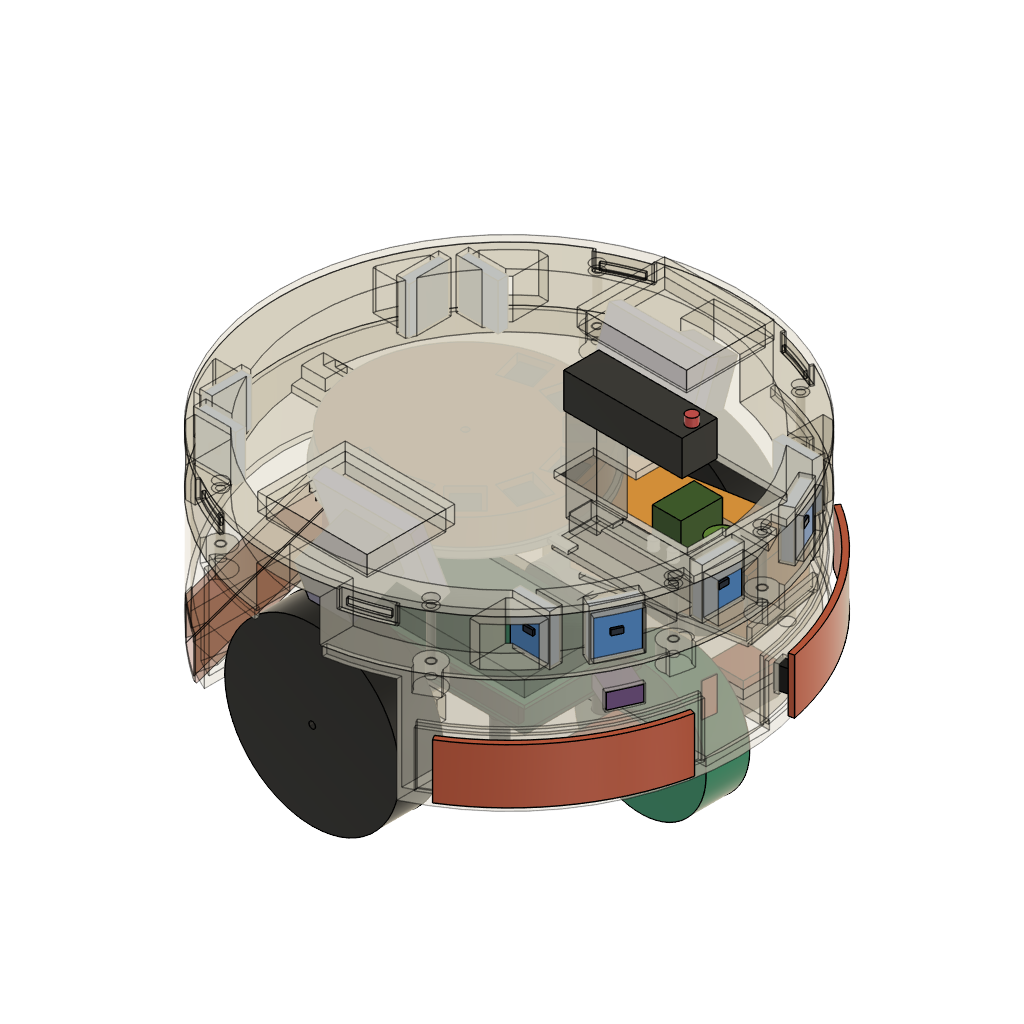
Theseus_V3_rev4 (Autodesk Fusion 360 design; units mm, degrees)
Autodesk Fusion 360 part; units mm, degrees
(part 1 of 3)
sketch "Tub shell sketch" plane through (0, 0, 0) normal (0, 0, 1) x (1, 0, 0) in component "Tub"
  circle A0 centre (0, 0) radius 105
extrude "Tub shell" add sketch "Tub shell sketch" along normal blind 52 from surface at 35 makes body 1 in component "Tub"
sketch "Cavity sketch" plane through (0, 0, 0) normal (0, 0, 1) x (1, 0, 0) in component "Tub"
  circle A0 centre (0, 0) radius 103
extrude "Cavity" cut sketch "Cavity sketch" along normal blind 53 from surface at 39 bodies 1 in component "Tub"
sketch "Rear chamfer sketch" plane through (0, 0, 0) normal (0, 1, 0) x (1, 0, 0) in component "Tub"
  line L0 (-65, -35) -> (-112, -56.15)
  line L1 (-112, -56.15) -> (-112, -29)
  line L2 (-112, -29) -> (-65, -29)
  line L3 (-65, -29) -> (-65, -35)
extrude "Rear chamfer" cut sketch "Rear chamfer sketch" along normal blind 220 from surface at -110 bodies 1 in component "Tub"
sketch "Wheel opening and arch L sketch" plane through (0, 0, 0) normal (0, 0, 1) x (1, 0, 0) in component "Tub"
  line L0 (-44, 69) -> (44, 69)
  line L1 (44, 69) -> (44, 108)
  line L2 (44, 108) -> (-44, 108)
  line L3 (-44, 108) -> (-44, 69)
extrude "Wheel opening and arch L" cut sketch "Wheel opening and arch L sketch" along normal blind 49 from surface at 34 bodies 1 in component "Tub"
sketch "Camera notch L sketch" plane through (0, 0, 0) normal (0, 0, 1) x (1, 0, 0) in component "Tub"
  line L0 (-11.9288, 69) -> (18.0712, 69)
  line L1 (18.0712, 69) -> (18.0712, 108)
  line L2 (18.0712, 108) -> (-11.9288, 108)
  line L3 (-11.9288, 108) -> (-11.9288, 69)
extrude "Camera notch L" cut sketch "Camera notch L sketch" along normal blind 6 from surface at 82 bodies 1 in component "Tub"
sketch "Motor seat L sketch" plane through (0, 0, 0) normal (0, 1, 0) x (1, 0, 0) in component "Tub"
  circle A0 centre (0, -40) radius 10.15
extrude "Motor seat L" cut sketch "Motor seat L sketch" along normal blind 51.5 from surface at 13 bodies 1 in component "Tub"
sketch "Shaft notch L sketch" plane through (0, 0, 0) normal (0, 1, 0) x (1, 0, 0) in component "Tub"
  line L0 (-3, -34.5) -> (3, -34.5)
  line L1 (3, -34.5) -> (3, -44.5)
  line L2 (3, -44.5) -> (-3, -44.5)
  line L3 (-3, -44.5) -> (-3, -34.5)
extrude "Shaft notch L" cut sketch "Shaft notch L sketch" along normal blind 4.5 from surface at 64.5 bodies 1 in component "Tub"
sketch "Plate slot L sketch" plane through (0, 0, 0) normal (0, 0, 1) x (1, 0, 0) in component "Tub"
  line L0 (-16, 60.5) -> (24.5, 60.5)
  line L1 (24.5, 60.5) -> (24.5, 64.5)
  line L2 (24.5, 64.5) -> (-16, 64.5)
  line L3 (-16, 64.5) -> (-16, 60.5)
extrude "Plate slot L" cut sketch "Plate slot L sketch" along normal blind 5 from surface at 34.5 bodies 1 in component "Tub"
sketch "Wheel opening and arch R sketch" plane through (0, 0, 0) normal (0, 0, 1) x (1, 0, 0) in component "Tub"
  line L0 (-44, -108) -> (44, -108)
  line L1 (44, -108) -> (44, -69)
  line L2 (44, -69) -> (-44, -69)
  line L3 (-44, -69) -> (-44, -108)
extrude "Wheel opening and arch R" cut sketch "Wheel opening and arch R sketch" along normal blind 49 from surface at 34 bodies 1 in component "Tub"
sketch "Camera notch R sketch" plane through (0, 0, 0) normal (0, 0, 1) x (1, 0, 0) in component "Tub"
  line L0 (-11.9288, -108) -> (18.0712, -108)
  line L1 (18.0712, -108) -> (18.0712, -69)
  line L2 (18.0712, -69) -> (-11.9288, -69)
  line L3 (-11.9288, -69) -> (-11.9288, -108)
extrude "Camera notch R" cut sketch "Camera notch R sketch" along normal blind 6 from surface at 82 bodies 1 in component "Tub"
sketch "Motor seat R sketch" plane through (0, 0, 0) normal (0, 1, 0) x (1, 0, 0) in component "Tub"
  circle A0 centre (0, -40) radius 10.15
extrude "Motor seat R" cut sketch "Motor seat R sketch" along normal blind 51.5 from surface at -64.5 bodies 1 in component "Tub"
sketch "Shaft notch R sketch" plane through (0, 0, 0) normal (0, 1, 0) x (1, 0, 0) in component "Tub"
  line L0 (-3, -34.5) -> (3, -34.5)
  line L1 (3, -34.5) -> (3, -44.5)
  line L2 (3, -44.5) -> (-3, -44.5)
  line L3 (-3, -44.5) -> (-3, -34.5)
extrude "Shaft notch R" cut sketch "Shaft notch R sketch" along normal blind 4.5 from surface at -69 bodies 1 in component "Tub"
sketch "Plate slot R sketch" plane through (0, 0, 0) normal (0, 0, 1) x (1, 0, 0) in component "Tub"
  line L0 (-16, -64.5) -> (24.5, -64.5)
  line L1 (24.5, -64.5) -> (24.5, -60.5)
  line L2 (24.5, -60.5) -> (-16, -60.5)
  line L3 (-16, -60.5) -> (-16, -64.5)
extrude "Plate slot R" cut sketch "Plate slot R sketch" along normal blind 5 from surface at 34.5 bodies 1 in component "Tub"
sketch "Omni bay 1 sketch" plane through (0, 0, 0) normal (0, 1, 0) x (1, 0, 0) in component "Tub"
  line L0 (38.5005, -29.8229) -> (38.4302, -42.3229)
  arc A0 (38.4302, -42.3229) -> (101.4292, -42.6771) centre (69.9297, -42.5) ccw
  line L1 (101.4292, -42.6771) -> (101.4995, -30.1771)
  arc A1 (101.4995, -30.1771) -> (38.5005, -29.8229) centre (70, -30) ccw
extrude "Omni bay 1" cut sketch "Omni bay 1 sketch" along normal blind 29 from surface at -11.5 bodies 1 in component "Tub"
sketch "Omni bay 2 sketch" plane through (0, 0, 0) normal (0, 1, 0) x (1, 0, 0) in component "Tub"
  line L0 (39.7548, -33.4597) -> (36.0099, -45.9597)
  arc A0 (36.0099, -45.9597) -> (96.3596, -64.0403) centre (66.1848, -55) ccw
  line L1 (96.3596, -64.0403) -> (100.1046, -51.5403)
  arc A1 (100.1046, -51.5403) -> (39.7548, -33.4597) centre (69.9297, -42.5) ccw
extrude "Omni bay 2" cut sketch "Omni bay 2 sketch" along normal blind 29 from surface at -11.5 bodies 1 in component "Tub"
sketch "Arm slot sketch" plane through (0, 0, 0) normal (0, 1, 0) x (1, 0, 0) in component "Tub"
  line L0 (26.569, -43.9283) -> (71.069, -37.9283)
  arc A0 (71.069, -37.9283) -> (68.931, -22.0717) centre (70, -30) ccw
  line L1 (68.931, -22.0717) -> (24.431, -28.0717)
  arc A1 (24.431, -28.0717) -> (26.569, -43.9283) centre (25.5, -36) ccw
extrude "Arm slot" cut sketch "Arm slot sketch" along normal blind 9 from surface at 8.5 bodies 1 in component "Tub"
sketch "Floor port FP hole sketch" plane through (0, 0, 0) normal (0, 0, 1) x (1, 0, 0) in component "Tub"
  line L0 (66.5, 23.5) -> (83.5, 23.5)
  line L1 (83.5, 23.5) -> (83.5, 40.5)
  line L2 (83.5, 40.5) -> (66.5, 40.5)
  line L3 (66.5, 40.5) -> (66.5, 23.5)
extrude "Floor port FP hole" cut sketch "Floor port FP hole sketch" along normal blind 6 from surface at 34 bodies 1 in component "Tub"
sketch "Silver module SM hole sketch" plane through (0, 0, 0) normal (0, 0, 1) x (1, 0, 0) in component "Tub"
  line L0 (64.5, -38.5) -> (85.5, -38.5)
  line L1 (85.5, -38.5) -> (85.5, -15.5)
  line L2 (85.5, -15.5) -> (64.5, -15.5)
  line L3 (64.5, -15.5) -> (64.5, -38.5)
extrude "Silver module SM hole" cut sketch "Silver module SM hole sketch" along normal blind 6 from surface at 34 bodies 1 in component "Tub"
sketch "Chute hole tool B left sketch" plane through (0, 0, 0) normal (0, 0, 1) x (1, 0, 0) in component "Tub"
  line L0 (-8.5, -8.5) -> (8.5, -8.5)
  line L1 (8.5, -8.5) -> (8.5, 8.5)
  line L2 (8.5, 8.5) -> (-8.5, 8.5)
  line L3 (-8.5, 8.5) -> (-8.5, -8.5)
extrude "Chute hole tool B left" add sketch "Chute hole tool B left sketch" along normal blind 79.2151 separate body makes body 2 in component "Tub"
move_body "Move1" bodies 2 to x (-0.977496, -0.210954, 0) y (-0.112564, 0.521586, 0.845741) z (-0.178413, 0.826708, -0.533594) at (-47.2943, 27.2943, 79.5) in component "Tub"
combine "Combine1" operation cut target body 1 tool bodies 2 in component "Tub"
sketch "Chute hole tool A right sketch" plane through (0, 0, 0) normal (0, 0, 1) x (1, 0, 0) in component "Tub"
  line L0 (-8.5, -8.5) -> (8.5, -8.5)
  line L1 (8.5, -8.5) -> (8.5, 8.5)
  line L2 (8.5, 8.5) -> (-8.5, 8.5)
  line L3 (-8.5, 8.5) -> (-8.5, -8.5)
extrude "Chute hole tool A right" add sketch "Chute hole tool A right sketch" along normal blind 79.2151 separate body makes body 3 in component "Tub"
move_body "Move2" bodies 3 to x (0.977496, -0.210954, 0) y (-0.112564, -0.521586, 0.845741) z (-0.178413, -0.826708, -0.533594) at (-47.2943, -27.2943, 79.5) in component "Tub"
combine "Combine2" operation cut target body 1 tool bodies 3 in component "Tub"
sketch "Bumper recess L sketch" plane through (0, 0, 0) normal (0, 0, 1) x (1, 0, 0) in component "Tub"
  arc A0 (106.949, 15.0307) -> (50.7029, 95.3583) centre (0, 0) ccw
  line L0 (50.7029, 95.3583) -> (48.5903, 91.3851)
  arc A1 (102.4927, 14.4044) -> (48.5903, 91.3851) centre (0, 0) ccw
  line L1 (102.4927, 14.4044) -> (106.949, 15.0307)
extrude "Bumper recess L" cut sketch "Bumper recess L sketch" along normal blind 25 from surface at 40 bodies 1 in component "Tub"
sketch "Bumper recess wall L sketch" plane through (0, 0, 0) normal (0, 0, 1) x (1, 0, 0) in component "Tub"
  arc A0 (102.1957, 14.3627) -> (48.4495, 91.1202) centre (0, 0) ccw
  line L0 (48.4495, 91.1202) -> (47.6514, 89.6192)
  arc A1 (100.5122, 14.1261) -> (47.6514, 89.6192) centre (0, 0) ccw
  line L1 (100.5122, 14.1261) -> (102.1957, 14.3627)
extrude "Bumper recess wall L" add sketch "Bumper recess wall L sketch" along normal blind 27 from surface at 39 bodies 1 in component "Tub"
sketch "Bumper switch pocket L sketch" plane through (0, 0, 0) normal (0, 0, 1) x (1, 0, 0) in component "Tub"
  line L0 (98.18, 21.6448) -> (101.576, 22.4916)
  line L1 (101.576, 22.4916) -> (100.2455, 27.8282)
  line L2 (100.2455, 27.8282) -> (96.8494, 26.9815)
  line L3 (96.8494, 26.9815) -> (98.18, 21.6448)
extrude "Bumper switch pocket L" cut sketch "Bumper switch pocket L sketch" along normal blind 12 from surface at 46.5 bodies 1 in component "Tub"
sketch "Bumper recess R sketch" plane through (0, 0, 0) normal (0, 0, 1) x (1, 0, 0) in component "Tub"
  arc A0 (50.7029, -95.3583) -> (106.949, -15.0307) centre (0, 0) ccw
  line L0 (106.949, -15.0307) -> (102.4927, -14.4044)
  arc A1 (48.5903, -91.3851) -> (102.4927, -14.4044) centre (0, 0) ccw
  line L1 (48.5903, -91.3851) -> (50.7029, -95.3583)
extrude "Bumper recess R" cut sketch "Bumper recess R sketch" along normal blind 25 from surface at 40 bodies 1 in component "Tub"
sketch "Bumper recess wall R sketch" plane through (0, 0, 0) normal (0, 0, 1) x (1, 0, 0) in component "Tub"
  arc A0 (48.4495, -91.1202) -> (102.1957, -14.3627) centre (0, 0) ccw
  line L0 (102.1957, -14.3627) -> (100.5122, -14.1261)
  arc A1 (47.6514, -89.6192) -> (100.5122, -14.1261) centre (0, 0) ccw
  line L1 (47.6514, -89.6192) -> (48.4495, -91.1202)
extrude "Bumper recess wall R" add sketch "Bumper recess wall R sketch" along normal blind 27 from surface at 39 bodies 1 in component "Tub"
sketch "Bumper switch pocket R sketch" plane through (0, 0, 0) normal (0, 0, 1) x (1, 0, 0) in component "Tub"
  line L0 (96.8494, -26.9815) -> (100.2455, -27.8282)
  line L1 (100.2455, -27.8282) -> (101.576, -22.4916)
  line L2 (101.576, -22.4916) -> (98.18, -21.6448)
  line L3 (98.18, -21.6448) -> (96.8494, -26.9815)
extrude "Bumper switch pocket R" cut sketch "Bumper switch pocket R sketch" along normal blind 12 from surface at 46.5 bodies 1 in component "Tub"
sketch "Insert boss +12 sketch" plane through (0, 0, 0) normal (0, 0, 1) x (1, 0, 0) in component "Tub"
  circle A0 centre (95.3694, 20.2714) radius 6
  line L0 (96.4089, 15.3807) -> (102.7669, 16.7321)
  line L1 (102.7669, 16.7321) -> (100.6878, 26.5136)
  line L2 (100.6878, 26.5136) -> (94.3298, 25.1621)
  line L3 (94.3298, 25.1621) -> (96.4089, 15.3807)
extrude "Insert boss +12" add sketch "Insert boss +12 sketch" along normal blind 10 from surface at 77 bodies 1 in component "Tub"
sketch "Insert boss +60 sketch" plane through (0, 0, 0) normal (0, 0, 1) x (1, 0, 0) in component "Tub"
  circle A0 centre (48.75, 84.4375) radius 6
  line L0 (53.0801, 81.9375) -> (56.3301, 87.5666)
  line L1 (56.3301, 87.5666) -> (47.6699, 92.5666)
  line L2 (47.6699, 92.5666) -> (44.4199, 86.9375)
  line L3 (44.4199, 86.9375) -> (53.0801, 81.9375)
extrude "Insert boss +60" add sketch "Insert boss +60 sketch" along normal blind 10 from surface at 77 bodies 1 in component "Tub"
sketch "Insert boss +118 sketch" plane through (0, 0, 0) normal (0, 0, 1) x (1, 0, 0) in component "Tub"
  circle A0 centre (-45.7735, 86.0874) radius 6
  line L0 (-41.3587, 88.4347) -> (-44.4103, 94.1739)
  line L1 (-44.4103, 94.1739) -> (-53.2398, 89.4792)
  line L2 (-53.2398, 89.4792) -> (-50.1882, 83.74)
  line L3 (-50.1882, 83.74) -> (-41.3587, 88.4347)
extrude "Insert boss +118" add sketch "Insert boss +118 sketch" along normal blind 10 from surface at 77 bodies 1 in component "Tub"
sketch "Insert boss -12 sketch" plane through (0, 0, 0) normal (0, 0, 1) x (1, 0, 0) in component "Tub"
  circle A0 centre (95.3694, -20.2714) radius 6
  line L0 (94.3298, -25.1621) -> (100.6878, -26.5136)
  line L1 (100.6878, -26.5136) -> (102.7669, -16.7321)
  line L2 (102.7669, -16.7321) -> (96.4089, -15.3807)
  line L3 (96.4089, -15.3807) -> (94.3298, -25.1621)
extrude "Insert boss -12" add sketch "Insert boss -12 sketch" along normal blind 10 from surface at 77 bodies 1 in component "Tub"
sketch "Insert boss -60 sketch" plane through (0, 0, 0) normal (0, 0, 1) x (1, 0, 0) in component "Tub"
  circle A0 centre (48.75, -84.4375) radius 6
  line L0 (44.4199, -86.9375) -> (47.6699, -92.5666)
  line L1 (47.6699, -92.5666) -> (56.3301, -87.5666)
  line L2 (56.3301, -87.5666) -> (53.0801, -81.9375)
  line L3 (53.0801, -81.9375) -> (44.4199, -86.9375)
extrude "Insert boss -60" add sketch "Insert boss -60 sketch" along normal blind 10 from surface at 77 bodies 1 in component "Tub"
sketch "Insert boss -118 sketch" plane through (0, 0, 0) normal (0, 0, 1) x (1, 0, 0) in component "Tub"
  circle A0 centre (-45.7735, -86.0874) radius 6
  line L0 (-50.1882, -83.74) -> (-53.2398, -89.4792)
  line L1 (-53.2398, -89.4792) -> (-44.4103, -94.1739)
  line L2 (-44.4103, -94.1739) -> (-41.3587, -88.4347)
  line L3 (-41.3587, -88.4347) -> (-50.1882, -83.74)
extrude "Insert boss -118" add sketch "Insert boss -118 sketch" along normal blind 10 from surface at 77 bodies 1 in component "Tub"
sketch "Cradle web rear L sketch" plane through (0, 0, 0) normal (0, 1, 0) x (1, 0, 0) in component "Tub"
  line L0 (-16, -38.5) -> (-3, -38.5)
  line L1 (-3, -38.5) -> (-3, -52)
  line L2 (-3, -52) -> (-16, -52)
  line L3 (-16, -52) -> (-16, -38.5)
extrude "Cradle web rear L" add sketch "Cradle web rear L sketch" along normal blind 2.5 from surface at 64.5 bodies 1 in component "Tub"
sketch "Cradle web front L sketch" plane through (0, 0, 0) normal (0, 1, 0) x (1, 0, 0) in component "Tub"
  line L0 (3, -38.5) -> (27.5, -38.5)
  line L1 (27.5, -38.5) -> (27.5, -52)
  line L2 (27.5, -52) -> (3, -52)
  line L3 (3, -52) -> (3, -38.5)
extrude "Cradle web front L" add sketch "Cradle web front L sketch" along normal blind 2.5 from surface at 64.5 bodies 1 in component "Tub"
sketch "Cradle ledge front L sketch" plane through (0, 0, 0) normal (0, 1, 0) x (1, 0, 0) in component "Tub"
  line L0 (10.6, -38.5) -> (27.5, -38.5)
  line L1 (27.5, -38.5) -> (27.5, -49)
  line L2 (27.5, -49) -> (10.6, -49)
  line L3 (10.6, -49) -> (10.6, -38.5)
extrude "Cradle ledge front L" add sketch "Cradle ledge front L sketch" along normal blind 4 from surface at 56.5 bodies 1 in component "Tub"
sketch "Cradle ledge rear L sketch" plane through (0, 0, 0) normal (0, 1, 0) x (1, 0, 0) in component "Tub"
  line L0 (-16, -38.5) -> (-10.6, -38.5)
  line L1 (-10.6, -38.5) -> (-10.6, -49)
  line L2 (-10.6, -49) -> (-16, -49)
  line L3 (-16, -49) -> (-16, -38.5)
extrude "Cradle ledge rear L" add sketch "Cradle ledge rear L sketch" along normal blind 4 from surface at 56.5 bodies 1 in component "Tub"
sketch "Cradle prong front L sketch" plane through (0, 0, 0) normal (0, 1, 0) x (1, 0, 0) in component "Tub"
  line L0 (13, -38.5) -> (13, -48)
  line L1 (13, -48) -> (8, -48)
  line L2 (8, -48) -> (7.8607, -46.5)
  line L3 (7.8607, -46.5) -> (8.544, -45.5714)
  line L4 (8.544, -45.5714) -> (9.0821, -44.6429)
  line L5 (9.0821, -44.6429) -> (9.4997, -43.7143)
  line L6 (9.4997, -43.7143) -> (9.8122, -42.7857)
  line L7 (9.8122, -42.7857) -> (10.0295, -41.8571)
  line L8 (10.0295, -41.8571) -> (10.1576, -40.9286)
  line L9 (10.1576, -40.9286) -> (10.2, -40)
  line L10 (10.2, -40) -> (10.6, -38.5)
  line L11 (10.6, -38.5) -> (13, -38.5)
extrude "Cradle prong front L" add sketch "Cradle prong front L sketch" along normal blind 32 from surface at 28.5 separate body makes body 4 in component "Tub"
sketch "Cradle prong rear L sketch" plane through (0, 0, 0) normal (0, 1, 0) x (1, 0, 0) in component "Tub"
  line L0 (-13, -38.5) -> (-13, -48)
  line L1 (-13, -48) -> (-8, -48)
  line L2 (-8, -48) -> (-7.8607, -46.5)
  line L3 (-7.8607, -46.5) -> (-8.544, -45.5714)
  line L4 (-8.544, -45.5714) -> (-9.0821, -44.6429)
  line L5 (-9.0821, -44.6429) -> (-9.4997, -43.7143)
  line L6 (-9.4997, -43.7143) -> (-9.8122, -42.7857)
  line L7 (-9.8122, -42.7857) -> (-10.0295, -41.8571)
  line L8 (-10.0295, -41.8571) -> (-10.1576, -40.9286)
  line L9 (-10.1576, -40.9286) -> (-10.2, -40)
  line L10 (-10.2, -40) -> (-10.6, -38.5)
  line L11 (-10.6, -38.5) -> (-13, -38.5)
extrude "Cradle prong rear L" add sketch "Cradle prong rear L sketch" along normal blind 32 from surface at 28.5 separate body makes body 5 in component "Tub"
sketch "Cradle web rear R sketch" plane through (0, 0, 0) normal (0, 1, 0) x (1, 0, 0) in component "Tub"
  line L0 (-16, -38.5) -> (-3, -38.5)
  line L1 (-3, -38.5) -> (-3, -52)
  line L2 (-3, -52) -> (-16, -52)
  line L3 (-16, -52) -> (-16, -38.5)
extrude "Cradle web rear R" add sketch "Cradle web rear R sketch" along normal blind 2.5 from surface at -67 bodies 1 in component "Tub"
sketch "Cradle web front R sketch" plane through (0, 0, 0) normal (0, 1, 0) x (1, 0, 0) in component "Tub"
  line L0 (3, -38.5) -> (27.5, -38.5)
  line L1 (27.5, -38.5) -> (27.5, -52)
  line L2 (27.5, -52) -> (3, -52)
  line L3 (3, -52) -> (3, -38.5)
extrude "Cradle web front R" add sketch "Cradle web front R sketch" along normal blind 2.5 from surface at -67 bodies 1 in component "Tub"
sketch "Cradle ledge front R sketch" plane through (0, 0, 0) normal (0, 1, 0) x (1, 0, 0) in component "Tub"
  line L0 (10.6, -38.5) -> (27.5, -38.5)
  line L1 (27.5, -38.5) -> (27.5, -49)
  line L2 (27.5, -49) -> (10.6, -49)
  line L3 (10.6, -49) -> (10.6, -38.5)
extrude "Cradle ledge front R" add sketch "Cradle ledge front R sketch" along normal blind 4 from surface at -60.5 bodies 1 in component "Tub"
sketch "Cradle ledge rear R sketch" plane through (0, 0, 0) normal (0, 1, 0) x (1, 0, 0) in component "Tub"
  line L0 (-16, -38.5) -> (-10.6, -38.5)
  line L1 (-10.6, -38.5) -> (-10.6, -49)
  line L2 (-10.6, -49) -> (-16, -49)
  line L3 (-16, -49) -> (-16, -38.5)
extrude "Cradle ledge rear R" add sketch "Cradle ledge rear R sketch" along normal blind 4 from surface at -60.5 bodies 1 in component "Tub"
sketch "Cradle prong front R sketch" plane through (0, 0, 0) normal (0, 1, 0) x (1, 0, 0) in component "Tub"
  line L0 (13, -38.5) -> (13, -48)
  line L1 (13, -48) -> (8, -48)
  line L2 (8, -48) -> (7.8607, -46.5)
  line L3 (7.8607, -46.5) -> (8.544, -45.5714)
  line L4 (8.544, -45.5714) -> (9.0821, -44.6429)
  line L5 (9.0821, -44.6429) -> (9.4997, -43.7143)
  line L6 (9.4997, -43.7143) -> (9.8122, -42.7857)
  line L7 (9.8122, -42.7857) -> (10.0295, -41.8571)
  line L8 (10.0295, -41.8571) -> (10.1576, -40.9286)
  line L9 (10.1576, -40.9286) -> (10.2, -40)
  line L10 (10.2, -40) -> (10.6, -38.5)
  line L11 (10.6, -38.5) -> (13, -38.5)
extrude "Cradle prong front R" add sketch "Cradle prong front R sketch" along normal blind 32 from surface at -60.5 separate body makes body 6 in component "Tub"
sketch "Cradle prong rear R sketch" plane through (0, 0, 0) normal (0, 1, 0) x (1, 0, 0) in component "Tub"
  line L0 (-13, -38.5) -> (-13, -48)
  line L1 (-13, -48) -> (-8, -48)
  line L2 (-8, -48) -> (-7.8607, -46.5)
  line L3 (-7.8607, -46.5) -> (-8.544, -45.5714)
  line L4 (-8.544, -45.5714) -> (-9.0821, -44.6429)
  line L5 (-9.0821, -44.6429) -> (-9.4997, -43.7143)
  line L6 (-9.4997, -43.7143) -> (-9.8122, -42.7857)
  line L7 (-9.8122, -42.7857) -> (-10.0295, -41.8571)
  line L8 (-10.0295, -41.8571) -> (-10.1576, -40.9286)
  line L9 (-10.1576, -40.9286) -> (-10.2, -40)
  line L10 (-10.2, -40) -> (-10.6, -38.5)
  line L11 (-10.6, -38.5) -> (-13, -38.5)
extrude "Cradle prong rear R" add sketch "Cradle prong rear R sketch" along normal blind 32 from surface at -60.5 separate body makes body 7 in component "Tub"
sketch "Tray leg sketch" plane through (0, 0, 0) normal (0, 0, 1) x (1, 0, 0) in component "Tub"
  circle A0 centre (66.4605, 60.5271) radius 3
extrude "Tray leg" add sketch "Tray leg sketch" along normal blind 11 from surface at 38.5 bodies 1 in component "Tub"
sketch "Tray leg sketch (1)" plane through (0, 0, 0) normal (0, 0, 1) x (1, 0, 0) in component "Tub"
  circle A0 centre (49.3095, 31.1019) radius 3
extrude "Tray leg (1)" add sketch "Tray leg sketch (1)" along normal blind 11 from surface at 38.5 bodies 1 in component "Tub"
sketch "Tray leg sketch (2)" plane through (0, 0, 0) normal (0, 0, 1) x (1, 0, 0) in component "Tub"
  circle A0 centre (32.7439, 44.4277) radius 3
extrude "Tray leg (2)" add sketch "Tray leg sketch (2)" along normal blind 11 from surface at 38.5 bodies 1 in component "Tub"
sketch "Battery tray sketch" plane through (0, 0, 0) normal (0, 0, 1) x (1, 0, 0) in component "Tub"
  line L0 (6.7594, 19.0297) -> (77.6656, 31.5324)
  line L1 (77.6656, 31.5324) -> (71.2406, 67.9703)
  line L2 (71.2406, 67.9703) -> (0.3344, 55.4676)
  line L3 (0.3344, 55.4676) -> (6.7594, 19.0297)
extrude "Battery tray" add sketch "Battery tray sketch" along normal blind 2 from surface at 49 bodies 1 in component "Tub"
sketch "Battery stop sketch" plane through (0, 0, 0) normal (0, 0, 1) x (1, 0, 0) in component "Tub"
  line L0 (77.1732, 31.4456) -> (79.1428, 31.7929)
  line L1 (79.1428, 31.7929) -> (72.7178, 68.2308)
  line L2 (72.7178, 68.2308) -> (70.7482, 67.8835)
  line L3 (70.7482, 67.8835) -> (77.1732, 31.4456)
extrude "Battery stop" add sketch "Battery stop sketch" along normal blind 6.5 from surface at 50.5 bodies 1 in component "Tub"
sketch "Battery tray notch sketch" plane through (0, 0, 0) normal (0, 0, 1) x (1, 0, 0) in component "Tub"
  line L0 (-12, 13) -> (12, 13)
  line L1 (12, 13) -> (12, 62)
  line L2 (12, 62) -> (-12, 62)
  line L3 (-12, 62) -> (-12, 13)
extrude "Battery tray notch" cut sketch "Battery tray notch sketch" along normal blind 4 from surface at 48 bodies 1 in component "Tub"
sketch "Insert hole +12 sketch" plane through (0, 0, 0) normal (0, 0, 1) x (1, 0, 0) in component "Tub"
  circle A0 centre (95.3694, 20.2714) radius 2
extrude "Insert hole +12" cut sketch "Insert hole +12 sketch" along normal blind 7 from surface at 81 bodies 1 in component "Tub"
sketch "Insert hole +60 sketch" plane through (0, 0, 0) normal (0, 0, 1) x (1, 0, 0) in component "Tub"
  circle A0 centre (48.75, 84.4375) radius 2
extrude "Insert hole +60" cut sketch "Insert hole +60 sketch" along normal blind 7 from surface at 81 bodies 1 in component "Tub"
sketch "Insert hole +118 sketch" plane through (0, 0, 0) normal (0, 0, 1) x (1, 0, 0) in component "Tub"
  circle A0 centre (-45.7735, 86.0874) radius 2
extrude "Insert hole +118" cut sketch "Insert hole +118 sketch" along normal blind 7 from surface at 81 bodies 1 in component "Tub"
sketch "Insert hole -12 sketch" plane through (0, 0, 0) normal (0, 0, 1) x (1, 0, 0) in component "Tub"
  circle A0 centre (95.3694, -20.2714) radius 2
extrude "Insert hole -12" cut sketch "Insert hole -12 sketch" along normal blind 7 from surface at 81 bodies 1 in component "Tub"
sketch "Insert hole -60 sketch" plane through (0, 0, 0) normal (0, 0, 1) x (1, 0, 0) in component "Tub"
  circle A0 centre (48.75, -84.4375) radius 2
extrude "Insert hole -60" cut sketch "Insert hole -60 sketch" along normal blind 7 from surface at 81 bodies 1 in component "Tub"
sketch "Insert hole -118 sketch" plane through (0, 0, 0) normal (0, 0, 1) x (1, 0, 0) in component "Tub"
  circle A0 centre (-45.7735, -86.0874) radius 2
extrude "Insert hole -118" cut sketch "Insert hole -118 sketch" along normal blind 7 from surface at 81 bodies 1 in component "Tub"
sketch "USB-C socket hole sketch" plane through (0, 0, 0) normal (0, 0, 1) x (1, 0, 0) in component "Tub"
  line L0 (87.5938, -46.6617) -> (95.8158, -50.3224)
  line L1 (95.8158, -50.3224) -> (101.5101, -37.5327)
  line L2 (101.5101, -37.5327) -> (93.2882, -33.8721)
  line L3 (93.2882, -33.8721) -> (87.5938, -46.6617)
extrude "USB-C socket hole" cut sketch "USB-C socket hole sketch" along normal blind 8 from surface at 71 bodies 1 in component "Tub"
sketch "Wheel L sketch" plane through (0, 0, 0) normal (0, 1, 0) x (1, 0, 0) in component "Wheel L"
  circle A0 centre (0, -40) radius 40
extrude "Wheel L" add sketch "Wheel L sketch" along normal blind 20 from surface at 70 separate body makes body 8 in component "Wheel L"
sketch "Shaft bore sketch" plane through (0, 0, 0) normal (0, 1, 0) x (1, 0, 0) in component "Wheel L"
  circle A0 centre (0, -40) radius 1.5
extrude "Shaft bore" cut sketch "Shaft bore sketch" along normal blind 22 from surface at 69 bodies 8 in component "Wheel L"
sketch "Encoder L sketch" plane through (0, 0, 0) normal (0, 1, 0) x (1, 0, 0) in component "Motor L"
  circle A0 centre (0, -40) radius 9
extrude "Encoder L" add sketch "Encoder L sketch" along normal blind 3 from surface at 14 separate body makes body 9 in component "Motor L"
sketch "Gearmotor L sketch" plane through (0, 0, 0) normal (0, 1, 0) x (1, 0, 0) in component "Motor L"
  circle A0 centre (0, -40) radius 10
extrude "Gearmotor L" add sketch "Gearmotor L sketch" along normal blind 44 from surface at 17 separate body makes body 10 in component "Motor L"
sketch "Motor shaft L sketch" plane through (0, 0, 0) normal (0, 1, 0) x (1, 0, 0) in component "Motor L"
  circle A0 centre (0, -40) radius 1.5
extrude "Motor shaft L" add sketch "Motor shaft L sketch" along normal blind 19 from surface at 61 separate body makes body 11 in component "Motor L"
sketch "Wheel R sketch" plane through (0, 0, 0) normal (0, 1, 0) x (1, 0, 0) in component "Wheel R"
  circle A0 centre (0, -40) radius 40
extrude "Wheel R" add sketch "Wheel R sketch" along normal blind 20 from surface at -90 separate body makes body 12 in component "Wheel R"
sketch "Shaft bore sketch (2)" plane through (0, 0, 0) normal (0, 1, 0) x (1, 0, 0) in component "Wheel R"
  circle A0 centre (0, -40) radius 1.5
extrude "Shaft bore'" cut sketch "Shaft bore sketch (2)" along normal blind 22 from surface at -91 bodies 12 in component "Wheel R"
sketch "Encoder R sketch" plane through (0, 0, 0) normal (0, 1, 0) x (1, 0, 0) in component "Motor R"
  circle A0 centre (0, -40) radius 9
extrude "Encoder R" add sketch "Encoder R sketch" along normal blind 3 from surface at -17 separate body makes body 13 in component "Motor R"
sketch "Gearmotor R sketch" plane through (0, 0, 0) normal (0, 1, 0) x (1, 0, 0) in component "Motor R"
  circle A0 centre (0, -40) radius 10
extrude "Gearmotor R" add sketch "Gearmotor R sketch" along normal blind 44 from surface at -61 separate body makes body 14 in component "Motor R"
sketch "Motor shaft R sketch" plane through (0, 0, 0) normal (0, 1, 0) x (1, 0, 0) in component "Motor R"
  circle A0 centre (0, -40) radius 1.5
extrude "Motor shaft R" add sketch "Motor shaft R sketch" along normal blind 19 from surface at -80 separate body makes body 15 in component "Motor R"
sketch "Face plate L sketch" plane through (0, 0, 0) normal (0, 1, 0) x (1, 0, 0) in component "Face plate L"
  line L0 (-15.5, -35.5) -> (23.5, -35.5)
  line L1 (23.5, -35.5) -> (23.5, -46)
  line L2 (23.5, -46) -> (15.5, -46)
  line L3 (15.5, -46) -> (15.5, -51)
  line L4 (15.5, -51) -> (-15.5, -51)
  line L5 (-15.5, -51) -> (-15.5, -35.5)
extrude "Face plate L" add sketch "Face plate L sketch" along normal blind 3 from surface at 61 separate body makes body 16 in component "Face plate L"
sketch "Shaft bore sketch (3)" plane through (0, 0, 0) normal (0, 1, 0) x (1, 0, 0) in component "Face plate L"
  circle A0 centre (0, -40) radius 2.2
extrude "Shaft bore''" cut sketch "Shaft bore sketch (3)" along normal blind 5 from surface at 60 bodies 16 in component "Face plate L"
sketch "Face plate R sketch" plane through (0, 0, 0) normal (0, 1, 0) x (1, 0, 0) in component "Face plate R"
  line L0 (-15.5, -35.5) -> (23.5, -35.5)
  line L1 (23.5, -35.5) -> (23.5, -46)
  line L2 (23.5, -46) -> (15.5, -46)
  line L3 (15.5, -46) -> (15.5, -51)
  line L4 (15.5, -51) -> (-15.5, -51)
  line L5 (-15.5, -51) -> (-15.5, -35.5)
extrude "Face plate R" add sketch "Face plate R sketch" along normal blind 3 from surface at -64 separate body makes body 17 in component "Face plate R"
sketch "Shaft bore sketch (4)" plane through (0, 0, 0) normal (0, 1, 0) x (1, 0, 0) in component "Face plate R"
  circle A0 centre (0, -40) radius 2.2
extrude "Shaft bore'''" cut sketch "Shaft bore sketch (4)" along normal blind 5 from surface at -65 bodies 17 in component "Face plate R"
sketch "Omni wheel sketch" plane through (0, 0, 0) normal (0, 1, 0) x (1, 0, 0) in component "Omni wheel"
  circle A0 centre (70, -30) radius 30
extrude "Omni wheel" add sketch "Omni wheel sketch" along normal blind 20 from surface at -10 separate body makes body 18 in component "Omni wheel"
sketch "Omni hub sketch" plane through (0, 0, 0) normal (0, 1, 0) x (1, 0, 0) in component "Omni wheel"
  circle A0 centre (70, -30) radius 10
extrude "Omni hub" add sketch "Omni hub sketch" along normal blind 22 from surface at -11 bodies 18 in component "Omni wheel"
sketch "Axle bore sketch" plane through (0, 0, 0) normal (0, 1, 0) x (1, 0, 0) in component "Omni wheel"
  circle A0 centre (70, -30) radius 2
extrude "Axle bore" cut sketch "Axle bore sketch" along normal blind 24 from surface at -12 bodies 18 in component "Omni wheel"
sketch "Arm plate sketch" plane through (0, 0, 0) normal (0, 1, 0) x (1, 0, 0) in component "Omni arm"
  line L0 (26.2349, -41.4507) -> (70.7349, -35.4507)
  arc A0 (70.7349, -35.4507) -> (69.2651, -24.5493) centre (70, -30) ccw
  line L1 (69.2651, -24.5493) -> (24.7651, -30.5493)
  arc A1 (24.7651, -30.5493) -> (26.2349, -41.4507) centre (25.5, -36) ccw
extrude "Arm plate" add sketch "Arm plate sketch" along normal blind 4 from surface at 11 separate body makes body 19 in component "Omni arm"
sketch "Pivot hole sketch" plane through (0, 0, 0) normal (0, 1, 0) x (1, 0, 0) in component "Omni arm"
  circle A0 centre (25.5, -36) radius 2
extrude "Pivot hole" cut sketch "Pivot hole sketch" along normal blind 6 from surface at 10 bodies 19 in component "Omni arm"
sketch "Axle hole sketch" plane through (0, 0, 0) normal (0, 1, 0) x (1, 0, 0) in component "Omni arm"
  circle A0 centre (70, -30) radius 2
extrude "Axle hole" cut sketch "Axle hole sketch" along normal blind 6 from surface at 10 bodies 19 in component "Omni arm"
sketch "Pivot pin sketch" plane through (0, 0, 0) normal (0, 1, 0) x (1, 0, 0) in component "Omni pins"
  circle A0 centre (25.5, -36) radius 2
extrude "Pivot pin" add sketch "Pivot pin sketch" along normal blind 8 from surface at 9 separate body makes body 20 in component "Omni pins"
sketch "Axle pin sketch" plane through (0, 0, 0) normal (0, 1, 0) x (1, 0, 0) in component "Omni pins"
  circle A0 centre (70, -30) radius 2
extrude "Axle pin" add sketch "Axle pin sketch" along normal blind 26.5 from surface at -10.5 separate body makes body 21 in component "Omni pins"
sketch "Rear nub sketch" plane through (0, 0, 0) normal (0, 0, 1) x (1, 0, 0) in component "Rear nub"
  circle A0 centre (-80, 0) radius 4
extrude "Rear nub" add sketch "Rear nub sketch" along normal blind 26 from surface at 20 separate body makes body 22 in component "Rear nub"
sketch "Seat on chamfer sketch" plane through (0, 0, 0) normal (0, 1, 0) x (1, 0, 0) in component "Rear nub"
  line L0 (-65, -35) -> (-112, -56.15)
  line L1 (-112, -56.15) -> (-112, -70)
  line L2 (-112, -70) -> (-65, -70)
  line L3 (-65, -70) -> (-65, -35)
extrude "Seat on chamfer" cut sketch "Seat on chamfer sketch" along normal blind 20 from surface at -10 bodies 22 in component "Rear nub"
sketch "Bumper plate L sketch" plane through (0, 0, 0) normal (0, 0, 1) x (1, 0, 0) in component "Bumper L"
  arc A0 (107.5962, 22.8703) -> (58.2911, 93.2853) centre (0, 0) ccw
  line L0 (58.2911, 93.2853) -> (56.9663, 91.1652)
  arc A1 (105.1509, 22.3505) -> (56.9663, 91.1652) centre (0, 0) ccw
  line L1 (105.1509, 22.3505) -> (107.5962, 22.8703)
extrude "Bumper plate L" add sketch "Bumper plate L sketch" along normal blind 25 from surface at 40 separate body makes body 23 in component "Bumper L"
sketch "Microswitch L sketch" plane through (0, 0, 0) normal (0, 0, 1) x (1, 0, 0) in component "Bumper switch L"
  line L0 (98.5442, 22.2509) -> (104.8511, 23.8234)
  line L1 (104.8511, 23.8234) -> (103.7625, 28.1898)
  line L2 (103.7625, 28.1898) -> (97.4555, 26.6173)
  line L3 (97.4555, 26.6173) -> (98.5442, 22.2509)
extrude "Microswitch L" add sketch "Microswitch L sketch" along normal blind 10 from surface at 47.5 separate body makes body 24 in component "Bumper switch L"
sketch "Bumper plate R sketch" plane through (0, 0, 0) normal (0, 0, 1) x (1, 0, 0) in component "Bumper R"
  arc A0 (58.2911, -93.2853) -> (107.5962, -22.8703) centre (0, 0) ccw
  line L0 (107.5962, -22.8703) -> (105.1509, -22.3505)
  arc A1 (56.9663, -91.1652) -> (105.1509, -22.3505) centre (0, 0) ccw
  line L1 (56.9663, -91.1652) -> (58.2911, -93.2853)
extrude "Bumper plate R" add sketch "Bumper plate R sketch" along normal blind 25 from surface at 40 separate body makes body 25 in component "Bumper R"
sketch "Microswitch R sketch" plane through (0, 0, 0) normal (0, 0, 1) x (1, 0, 0) in component "Bumper switch R"
  line L0 (97.4555, -26.6173) -> (103.7625, -28.1898)
  line L1 (103.7625, -28.1898) -> (104.8511, -23.8234)
  line L2 (104.8511, -23.8234) -> (98.5442, -22.2509)
  line L3 (98.5442, -22.2509) -> (97.4555, -26.6173)
extrude "Microswitch R" add sketch "Microswitch R sketch" along normal blind 10 from surface at 47.5 separate body makes body 26 in component "Bumper switch R"
sketch "Frame ring sketch" plane through (0, 0, 0) normal (0, 0, 1) x (1, 0, 0) in component "Upper frame"
  circle A0 centre (0, 0) radius 105
  circle A1 centre (0, 0) radius 90
extrude "Frame ring" add sketch "Frame ring sketch" along normal blind 25 from surface at 87 separate body makes body 27 in component "Upper frame"
sketch "Bridge web sketch" plane through (0, 0, 0) normal (0, 0, 1) x (1, 0, 0) in component "Upper frame"
  line L0 (32, -12.5) -> (92, -12.5)
  line L1 (92, -12.5) -> (92, 12.5)
  line L2 (92, 12.5) -> (32, 12.5)
  line L3 (32, 12.5) -> (32, -12.5)
extrude "Bridge web" add sketch "Bridge web sketch" along normal blind 3 from surface at 87 bodies 27 in component "Upper frame"
sketch "Bridge rib sketch" plane through (0, 0, 0) normal (0, 0, 1) x (1, 0, 0) in component "Upper frame"
  line L0 (32.5, -5) -> (90.5, -5)
  line L1 (90.5, -5) -> (90.5, 5)
  line L2 (90.5, 5) -> (32.5, 5)
  line L3 (32.5, 5) -> (32.5, -5)
extrude "Bridge rib" add sketch "Bridge rib sketch" along normal blind 8.5 from surface at 89.5 bodies 27 in component "Upper frame"
sketch "Spoke web sketch" plane through (0, 0, 0) normal (0, 0, 1) x (1, 0, 0) in component "Upper frame"
  line L0 (-92, -10) -> (-72, -10)
  line L1 (-72, -10) -> (-72, 10)
  line L2 (-72, 10) -> (-92, 10)
  line L3 (-92, 10) -> (-92, -10)
extrude "Spoke web" add sketch "Spoke web sketch" along normal blind 3 from surface at 87 bodies 27 in component "Upper frame"
sketch "Spoke rib sketch" plane through (0, 0, 0) normal (0, 0, 1) x (1, 0, 0) in component "Upper frame"
  line L0 (-92, -5) -> (-79, -5)
  line L1 (-79, -5) -> (-79, 5)
  line L2 (-79, 5) -> (-92, 5)
  line L3 (-92, 5) -> (-92, -5)
extrude "Spoke rib" add sketch "Spoke rib sketch" along normal blind 5.5 from surface at 89.5 bodies 27 in component "Upper frame"
sketch "Control deck sketch" plane through (0, 0, 0) normal (0, 0, 1) x (1, 0, 0) in component "Upper frame"
  line L0 (52, -12.5) -> (91.5, -12.5)
  line L1 (91.5, -12.5) -> (91.5, 36)
  line L2 (91.5, 36) -> (52, 36)
  line L3 (52, 36) -> (52, -12.5)
extrude "Control deck" add sketch "Control deck sketch" along normal blind 3 from surface at 87 bodies 27 in component "Upper frame"
sketch "Handle post sketch" plane through (0, 0, 0) normal (0, 0, 1) x (1, 0, 0) in component "Upper frame"
  line L0 (33, -7) -> (47, -7)
  line L1 (47, -7) -> (47, 7)
  line L2 (47, 7) -> (33, 7)
  line L3 (33, 7) -> (33, -7)
extrude "Handle post" add sketch "Handle post sketch" along normal blind 43 from surface at 97 bodies 27 in component "Upper frame"
sketch "Seat rebate 0 sketch" plane through (0, 0, 0) normal (0, 0, 1) x (1, 0, 0) in component "Upper frame"
  line L0 (31.5, 8) -> (39.5, 8)
  line L1 (39.5, 8) -> (39.5, 13)
  line L2 (39.5, 13) -> (31.5, 13)
  line L3 (31.5, 13) -> (31.5, 8)
extrude "Seat rebate 0" cut sketch "Seat rebate 0 sketch" along normal blind 2.5 from surface at 88.5 bodies 27 in component "Upper frame"
sketch "Seat rebate 1 sketch" plane through (0, 0, 0) normal (0, 0, 1) x (1, 0, 0) in component "Upper frame"
  line L0 (31.5, -13) -> (39.5, -13)
  line L1 (39.5, -13) -> (39.5, -8)
  line L2 (39.5, -8) -> (31.5, -8)
  line L3 (31.5, -8) -> (31.5, -13)
extrude "Seat rebate 1" cut sketch "Seat rebate 1 sketch" along normal blind 2.5 from surface at 88.5 bodies 27 in component "Upper frame"
sketch "Seat rebate 2 sketch" plane through (0, 0, 0) normal (0, 0, 1) x (1, 0, 0) in component "Upper frame"
  line L0 (-75.5, -5.5) -> (-71.5, -5.5)
  line L1 (-71.5, -5.5) -> (-71.5, 5.5)
  line L2 (-71.5, 5.5) -> (-75.5, 5.5)
  line L3 (-75.5, 5.5) -> (-75.5, -5.5)
extrude "Seat rebate 2" cut sketch "Seat rebate 2 sketch" along normal blind 2.5 from surface at 88.5 bodies 27 in component "Upper frame"
sketch "Screw hole +12 sketch" plane through (0, 0, 0) normal (0, 0, 1) x (1, 0, 0) in component "Upper frame"
  circle A0 centre (95.3694, 20.2714) radius 1.65
extrude "Screw hole +12" cut sketch "Screw hole +12 sketch" along normal blind 27 from surface at 86 bodies 27 in component "Upper frame"
sketch "Screw counterbore +12 sketch" plane through (0, 0, 0) normal (0, 0, 1) x (1, 0, 0) in component "Upper frame"
  circle A0 centre (95.3694, 20.2714) radius 3
extrude "Screw counterbore +12" cut sketch "Screw counterbore +12 sketch" along normal blind 4 from surface at 109 bodies 27 in component "Upper frame"
sketch "Screw hole +60 sketch" plane through (0, 0, 0) normal (0, 0, 1) x (1, 0, 0) in component "Upper frame"
  circle A0 centre (48.75, 84.4375) radius 1.65
extrude "Screw hole +60" cut sketch "Screw hole +60 sketch" along normal blind 27 from surface at 86 bodies 27 in component "Upper frame"
sketch "Screw counterbore +60 sketch" plane through (0, 0, 0) normal (0, 0, 1) x (1, 0, 0) in component "Upper frame"
  circle A0 centre (48.75, 84.4375) radius 3
extrude "Screw counterbore +60" cut sketch "Screw counterbore +60 sketch" along normal blind 4 from surface at 109 bodies 27 in component "Upper frame"
sketch "Screw hole +118 sketch" plane through (0, 0, 0) normal (0, 0, 1) x (1, 0, 0) in component "Upper frame"
  circle A0 centre (-45.7735, 86.0874) radius 1.65
extrude "Screw hole +118" cut sketch "Screw hole +118 sketch" along normal blind 27 from surface at 86 bodies 27 in component "Upper frame"
sketch "Screw counterbore +118 sketch" plane through (0, 0, 0) normal (0, 0, 1) x (1, 0, 0) in component "Upper frame"
  circle A0 centre (-45.7735, 86.0874) radius 3
extrude "Screw counterbore +118" cut sketch "Screw counterbore +118 sketch" along normal blind 4 from surface at 109 bodies 27 in component "Upper frame"
sketch "Screw hole -12 sketch" plane through (0, 0, 0) normal (0, 0, 1) x (1, 0, 0) in component "Upper frame"
  circle A0 centre (95.3694, -20.2714) radius 1.65
extrude "Screw hole -12" cut sketch "Screw hole -12 sketch" along normal blind 27 from surface at 86 bodies 27 in component "Upper frame"
sketch "Screw counterbore -12 sketch" plane through (0, 0, 0) normal (0, 0, 1) x (1, 0, 0) in component "Upper frame"
  circle A0 centre (95.3694, -20.2714) radius 3
extrude "Screw counterbore -12" cut sketch "Screw counterbore -12 sketch" along normal blind 4 from surface at 109 bodies 27 in component "Upper frame"
sketch "Screw hole -60 sketch" plane through (0, 0, 0) normal (0, 0, 1) x (1, 0, 0) in component "Upper frame"
  circle A0 centre (48.75, -84.4375) radius 1.65
extrude "Screw hole -60" cut sketch "Screw hole -60 sketch" along normal blind 27 from surface at 86 bodies 27 in component "Upper frame"
sketch "Screw counterbore -60 sketch" plane through (0, 0, 0) normal (0, 0, 1) x (1, 0, 0) in component "Upper frame"
  circle A0 centre (48.75, -84.4375) radius 3
extrude "Screw counterbore -60" cut sketch "Screw counterbore -60 sketch" along normal blind 4 from surface at 109 bodies 27 in component "Upper frame"
sketch "Screw hole -118 sketch" plane through (0, 0, 0) normal (0, 0, 1) x (1, 0, 0) in component "Upper frame"
  circle A0 centre (-45.7735, -86.0874) radius 1.65
extrude "Screw hole -118" cut sketch "Screw hole -118 sketch" along normal blind 27 from surface at 86 bodies 27 in component "Upper frame"
sketch "Screw counterbore -118 sketch" plane through (0, 0, 0) normal (0, 0, 1) x (1, 0, 0) in component "Upper frame"
  circle A0 centre (-45.7735, -86.0874) radius 3
extrude "Screw counterbore -118" cut sketch "Screw counterbore -118 sketch" along normal blind 4 from surface at 109 bodies 27 in component "Upper frame"
sketch "Hook rebate +71 sketch" plane through (0, 0, 0) normal (0, 0, 1) x (1, 0, 0) in component "Upper frame"
  arc A0 (44.7975, 96.0686) -> (23.8448, 103.2832) centre (0, 0) ccw
  line L0 (23.8448, 103.2832) -> (23.2599, 100.7499)
  arc A1 (43.6987, 93.7122) -> (23.2599, 100.7499) centre (0, 0) ccw
  line L1 (43.6987, 93.7122) -> (44.7975, 96.0686)
extrude "Hook rebate +71" cut sketch "Hook rebate +71 sketch" along normal blind 9 from surface at 104 bodies 27 in component "Upper frame"
sketch "Hook groove +71 sketch" plane through (0, 0, 0) normal (0, 0, 1) x (1, 0, 0) in component "Upper frame"
  arc A0 (41.2705, 94.9157) -> (25.9143, 100.2033) centre (0, 0) ccw
  line L0 (25.9143, 100.2033) -> (25.6389, 99.1383)
  arc A1 (40.8319, 93.907) -> (25.6389, 99.1383) centre (0, 0) ccw
  line L1 (40.8319, 93.907) -> (41.2705, 94.9157)
extrude "Hook groove +71" cut sketch "Hook groove +71 sketch" along normal blind 3 from surface at 105.5 bodies 27 in component "Upper frame"
sketch "Hook rebate +114 sketch" plane through (0, 0, 0) normal (0, 0, 1) x (1, 0, 0) in component "Upper frame"
  arc A0 (-32.7558, 100.812) -> (-53, 91.7987) centre (0, 0) ccw
  line L0 (-53, 91.7987) -> (-51.7, 89.547)
  arc A1 (-31.9524, 98.3392) -> (-51.7, 89.547) centre (0, 0) ccw
  line L1 (-31.9524, 98.3392) -> (-32.7558, 100.812)
extrude "Hook rebate +114" cut sketch "Hook rebate +114 sketch" along normal blind 9 from surface at 104 bodies 27 in component "Upper frame"
sketch "Hook groove +114 sketch" plane through (0, 0, 0) normal (0, 0, 1) x (1, 0, 0) in component "Upper frame"
  arc A0 (-34.549, 97.5634) -> (-49.3859, 90.9576) centre (0, 0) ccw
  line L0 (-49.3859, 90.9576) -> (-48.8611, 89.9909)
  arc A1 (-34.1818, 96.5265) -> (-48.8611, 89.9909) centre (0, 0) ccw
  line L1 (-34.1818, 96.5265) -> (-34.549, 97.5634)
extrude "Hook groove +114" cut sketch "Hook groove +114 sketch" along normal blind 3 from surface at 105.5 bodies 27 in component "Upper frame"
sketch "Hook rebate -71 sketch" plane through (0, 0, 0) normal (0, 0, 1) x (1, 0, 0) in component "Upper frame"
  arc A0 (23.8448, -103.2832) -> (44.7975, -96.0686) centre (0, 0) ccw
  line L0 (44.7975, -96.0686) -> (43.6987, -93.7122)
  arc A1 (23.2599, -100.7499) -> (43.6987, -93.7122) centre (0, 0) ccw
  line L1 (23.2599, -100.7499) -> (23.8448, -103.2832)
extrude "Hook rebate -71" cut sketch "Hook rebate -71 sketch" along normal blind 9 from surface at 104 bodies 27 in component "Upper frame"
sketch "Hook groove -71 sketch" plane through (0, 0, 0) normal (0, 0, 1) x (1, 0, 0) in component "Upper frame"
  arc A0 (25.9143, -100.2033) -> (41.2705, -94.9157) centre (0, 0) ccw
  line L0 (41.2705, -94.9157) -> (40.8319, -93.907)
  arc A1 (25.6389, -99.1383) -> (40.8319, -93.907) centre (0, 0) ccw
  line L1 (25.6389, -99.1383) -> (25.9143, -100.2033)
extrude "Hook groove -71" cut sketch "Hook groove -71 sketch" along normal blind 3 from surface at 105.5 bodies 27 in component "Upper frame"
sketch "Hook rebate -114 sketch" plane through (0, 0, 0) normal (0, 0, 1) x (1, 0, 0) in component "Upper frame"
  arc A0 (-53, -91.7987) -> (-32.7558, -100.812) centre (0, 0) ccw
  line L0 (-32.7558, -100.812) -> (-31.9524, -98.3392)
  arc A1 (-51.7, -89.547) -> (-31.9524, -98.3392) centre (0, 0) ccw
  line L1 (-51.7, -89.547) -> (-53, -91.7987)
extrude "Hook rebate -114" cut sketch "Hook rebate -114 sketch" along normal blind 9 from surface at 104 bodies 27 in component "Upper frame"
sketch "Hook groove -114 sketch" plane through (0, 0, 0) normal (0, 0, 1) x (1, 0, 0) in component "Upper frame"
  arc A0 (-49.3859, -90.9576) -> (-34.549, -97.5634) centre (0, 0) ccw
  line L0 (-34.549, -97.5634) -> (-34.1818, -96.5265)
  arc A1 (-48.8611, -89.9909) -> (-34.1818, -96.5265) centre (0, 0) ccw
  line L1 (-48.8611, -89.9909) -> (-49.3859, -90.9576)
extrude "Hook groove -114" cut sketch "Hook groove -114 sketch" along normal blind 3 from surface at 105.5 bodies 27 in component "Upper frame"
sketch "Pocket F sketch" plane through (0, 0, 0) normal (0, 0, 1) x (1, 0, 0) in component "Upper frame"
  line L0 (92.15, 9.6) -> (97.85, 9.6)
  line L1 (97.85, 9.6) -> (97.85, -9.6)
  line L2 (97.85, -9.6) -> (92.15, -9.6)
  line L3 (92.15, -9.6) -> (92.15, 9.6)
extrude "Pocket F" cut sketch "Pocket F sketch" along normal blind 24 from surface at 89 bodies 27 in component "Upper frame"
sketch "Beam F sketch" plane through (0, 0, 0) normal (0, 0, 1) x (1, 0, 0) in component "Upper frame"
  line L0 (95, 9) -> (108, 9)
  line L1 (108, 9) -> (108, -9)
  line L2 (108, -9) -> (95, -9)
  line L3 (95, -9) -> (95, 9)
extrude "Beam F" cut sketch "Beam F sketch" along normal blind 18 from surface at 91 bodies 27 in component "Upper frame"
sketch "Pocket FL sketch" plane through (0, 0, 0) normal (0, 0, 1) x (1, 0, 0) in component "Upper frame"
  line L0 (83.0844, 49.3353) -> (88.2503, 51.7442)
  line L1 (88.2503, 51.7442) -> (96.3646, 34.3431)
  line L2 (96.3646, 34.3431) -> (91.1986, 31.9342)
  line L3 (91.1986, 31.9342) -> (83.0844, 49.3353)
extrude "Pocket FL" cut sketch "Pocket FL sketch" along normal blind 24 from surface at 89 bodies 27 in component "Upper frame"
sketch "Beam FL sketch" plane through (0, 0, 0) normal (0, 0, 1) x (1, 0, 0) in component "Upper frame"
  line L0 (85.9209, 49.996) -> (94.0777, 53.7995)
  line L1 (94.0777, 53.7995) -> (101.6848, 37.486)
  line L2 (101.6848, 37.486) -> (93.528, 33.6824)
  line L3 (93.528, 33.6824) -> (85.9209, 49.996)
extrude "Beam FL" cut sketch "Beam FL sketch" along normal blind 18 from surface at 91 bodies 27 in component "Upper frame"
sketch "Pocket FR sketch" plane through (0, 0, 0) normal (0, 0, 1) x (1, 0, 0) in component "Upper frame"
  line L0 (91.1986, -31.9342) -> (96.3646, -34.3431)
  line L1 (96.3646, -34.3431) -> (88.2503, -51.7442)
  line L2 (88.2503, -51.7442) -> (83.0844, -49.3353)
  line L3 (83.0844, -49.3353) -> (91.1986, -31.9342)
extrude "Pocket FR" cut sketch "Pocket FR sketch" along normal blind 24 from surface at 89 bodies 27 in component "Upper frame"
sketch "Beam FR sketch" plane through (0, 0, 0) normal (0, 0, 1) x (1, 0, 0) in component "Upper frame"
  line L0 (93.528, -33.6824) -> (101.6848, -37.486)
  line L1 (101.6848, -37.486) -> (94.0777, -53.7995)
  line L2 (94.0777, -53.7995) -> (85.9209, -49.996)
  line L3 (85.9209, -49.996) -> (93.528, -33.6824)
extrude "Beam FR" cut sketch "Beam FR sketch" along normal blind 18 from surface at 91 bodies 27 in component "Upper frame"
sketch "Pocket SFL sketch" plane through (0, 0, 0) normal (0, 0, 1) x (1, 0, 0) in component "Upper frame"
  line L0 (62.2, 57.15) -> (62.2, 62.85)
  line L1 (62.2, 62.85) -> (81.4, 62.85)
  line L2 (81.4, 62.85) -> (81.4, 57.15)
  line L3 (81.4, 57.15) -> (62.2, 57.15)
extrude "Pocket SFL" cut sketch "Pocket SFL sketch" along normal blind 24 from surface at 89 bodies 27 in component "Upper frame"
sketch "Beam SFL sketch" plane through (0, 0, 0) normal (0, 0, 1) x (1, 0, 0) in component "Upper frame"
  line L0 (62.8, 60) -> (62.8, 80.6769)
  line L1 (62.8, 80.6769) -> (80.8, 80.6769)
  line L2 (80.8, 80.6769) -> (80.8, 60)
  line L3 (80.8, 60) -> (62.8, 60)
extrude "Beam SFL" cut sketch "Beam SFL sketch" along normal blind 18 from surface at 91 bodies 27 in component "Upper frame"
sketch "Pocket SFR sketch" plane through (0, 0, 0) normal (0, 0, 1) x (1, 0, 0) in component "Upper frame"
  line L0 (81.4, -57.15) -> (81.4, -62.85)
  line L1 (81.4, -62.85) -> (62.2, -62.85)
  line L2 (62.2, -62.85) -> (62.2, -57.15)
  line L3 (62.2, -57.15) -> (81.4, -57.15)
extrude "Pocket SFR" cut sketch "Pocket SFR sketch" along normal blind 24 from surface at 89 bodies 27 in component "Upper frame"
sketch "Beam SFR sketch" plane through (0, 0, 0) normal (0, 0, 1) x (1, 0, 0) in component "Upper frame"
  line L0 (80.8, -60) -> (80.8, -80.6769)
  line L1 (80.8, -80.6769) -> (62.8, -80.6769)
  line L2 (62.8, -80.6769) -> (62.8, -60)
  line L3 (62.8, -60) -> (80.8, -60)
extrude "Beam SFR" cut sketch "Beam SFR sketch" along normal blind 18 from surface at 91 bodies 27 in component "Upper frame"